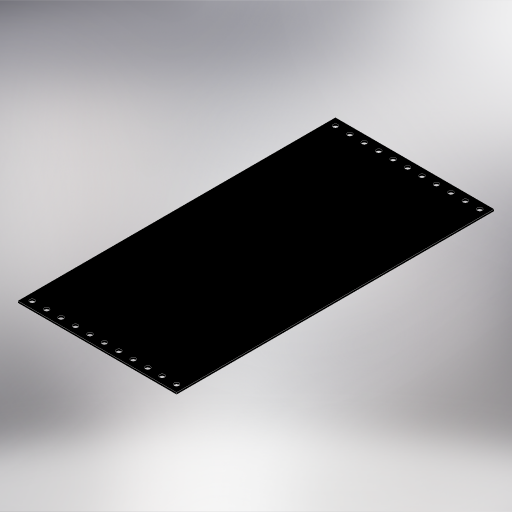
# Autodesk Inventor part: Blocker
Saved by Autodesk Inventor 2024 (Build 280153000, 153)
## iProperties
Created: 2023-10-21
Part Number: Blocker
Material: Generic
Document SubType Name: Modeling
Designer: aaron
Density: 1 g/cm^3
Appearance: Default
Author: aaron
Autodesk Inventor part; units mm, degrees
ref_plane "YZ Plane" through (0, 0, 0) normal (1, 0, 0) x (0, 1, 0)
ref_plane "XZ Plane" through (0, 0, 0) normal (0, 1, 0) x (-1, 0, 0)
ref_plane "XY Plane" through (0, 0, 0) normal (0, 0, 1) x (1, 0, 0)
sketch "Sketch1" plane through (0, 0, 0) normal (0, 1, 0) x (-1, 0, 0)
  line L0 (-69.85, -139.7) -> (69.85, -139.7)
  line L1 (69.85, -139.7) -> (69.85, 139.7)
  line L2 (69.85, 139.7) -> (-69.85, 139.7)
  line L3 (-69.85, 139.7) -> (-69.85, -139.7)
  line L4 (-69.85, -139.7) -> (69.85, 139.7) construction
  line L5 (69.85, -139.7) -> (-69.85, 139.7) construction
  point P0 (0, 0)
  dimension "d0" = 139.7
  dimension "d1" = 279.4
  constraints: 12 end point, 2 midpoint, 2 parallel, 1 horizontal, 1 perpendicular
  measures "d0" distance of L2.end L1.end
  measures "d1" distance of L1.end L0.end
extrude "Extrusion1" add sketch "Sketch1" along normal blind 1.5875
sketch "Sketch2" plane through (0, 1.5875, 0) normal (0, 1, 0) x (1, 0, 0)
  circle A0 centre (-63.5, 133.35) radius 2.1082
  line L0 (-69.85, 139.7) -> (-69.85, -139.7) projected
  line L1 (69.85, 139.7) -> (-69.85, 139.7) projected
  point P0 (0, 0)
  dimension "d4" = 4.2164
  dimension "d5" = 6.35
  dimension "d6" = 6.35
  constraints: 1 centre point
  measures "d4" diameter of A0
  measures "d5" distance from line of L0 A0.centre
  measures "d6" distance from line of L1 A0.centre
extrude "Extrusion2" cut sketch "Sketch2" against normal blind 1.5875
pattern_linear "Rectangular Pattern1" count 11 spacing 12.7 along (1, 0, 0) count 2 spacing 266.7 along (0, 0, 1) of "Extrusion2"
body "Solid1"
